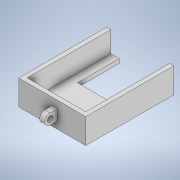
# Autodesk Inventor part: CAM04
Saved by Autodesk Inventor 2020.3 (Build 243373000, 373)
## iProperties
Created: 2021-05-24
Part Number: CAM04
Material: Generic
Document SubType Name: Modeling
Designer: patry
Density: 1 g/cm^3
Appearance: Default
Author: patry
Autodesk Inventor part; units mm, degrees
ref_plane "YZ Plane" through (0, 0, 0) normal (1, 0, 0) x (0, 1, 0)
ref_plane "XZ Plane" through (0, 0, 0) normal (0, 1, 0) x (-1, 0, 0)
ref_plane "XY Plane" through (0, 0, 0) normal (0, 0, 1) x (1, 0, 0)
sketch "Sketch1" plane through (0, 0, 0) normal (0, 1, 0) x (-1, 0, 0)
  line L0 (0, 0) -> (-32, 0)
  line L1 (-32, 0) -> (-32, 42)
  line L2 (-32, 42) -> (0, 42)
  line L3 (0, 42) -> (0, 0)
  dimension "d0" = 32
  dimension "d1" = 42
  constraints: 8 end point, 2 parallel, 1 horizontal, 1 perpendicular
  measures "d0" distance of L1.end L2.end
  measures "d1" distance of L0.end L1.end
extrude "Extrusion1" add sketch "Sketch1" along normal blind 2
sketch "Sketch2" plane through (0, 2, 0) normal (0, 1, 0) x (1, 0, 0)
  line L0 (0, -42) -> (32, -42) projected
  line L1 (0, 0) -> (32, 0)
  line L2 (32, 0) -> (32, -42)
  line L3 (32, -42) -> (0, -42)
  line L4 (0, -42) -> (0, 0)
  line L5 (0, 0) -> (0, -42) projected
  line L6 (0, 0) -> (2, 0)
  line L7 (2, 0) -> (2, -2)
  line L8 (2, -2) -> (0, -2)
  line L9 (0, -2) -> (0, 0)
  line L10 (32, -42) -> (30, -42)
  line L11 (30, -42) -> (30, -40)
  line L12 (30, -40) -> (32, -40)
  line L13 (32, -40) -> (32, -42)
  line L14 (30, -40) -> (2, -40)
  line L15 (2, -40) -> (2, -2)
  line L16 (2, -2) -> (30, -2)
  line L17 (30, -2) -> (30, -40)
  line L18 (32, -42) -> (32, 0) projected
  line L19 (30, -2) -> (32, -2)
  line L20 (32, -2) -> (32, 0)
  line L21 (32, 0) -> (30, 0)
  line L22 (30, 0) -> (30, -2)
  dimension "d4" = 2
  dimension "d5" = 2
  dimension "d6" = 2
  dimension "d7" = 2
  constraints: 40 end point, 10 parallel, 5 horizontal, 5 perpendicular
  measures "d4" distance of L7.end L8.end
  measures "d5" distance of L6.end L7.end
  measures "d6" distance of L11.end L12.end
  measures "d7" distance of L10.end L11.end
extrude "Extrusion2" add sketch "Sketch2" along normal blind 10 contours L4 L8 L15 L14 L11 L0 | L11 L12 L2 L0 | L4 L1 L7 L8 | L17 L19 L2 L12 | L22 L1 L2 L19
sketch "Sketch3" plane through (0, 2, 0) normal (0, 1, 0) x (1, 0, 0)
  line L0 (30, 0) -> (2, 0) projected
  line L1 (30, 0) -> (30, -40) projected
  line L2 (2, 0) -> (30, 0)
  line L3 (30, 0) -> (30, -40)
  line L4 (30, -40) -> (2, -40)
  line L5 (2, -40) -> (2, 0)
  line L6 (2, 0) -> (6, 0)
  line L7 (6, 0) -> (6, -4)
  line L8 (6, -4) -> (2, -4)
  line L9 (2, -4) -> (2, 0)
  line L10 (30, 0) -> (26, 0)
  line L11 (26, 0) -> (26, -4)
  line L12 (26, -4) -> (30, -4)
  line L13 (30, -4) -> (30, 0)
  line L14 (6, 0) -> (26, 0)
  line L15 (26, 0) -> (26, -20)
  line L16 (26, -20) -> (6, -20)
  line L17 (6, -20) -> (6, 0)
  point P0 (0, 0)
  dimension "d10" = 4
  dimension "d11" = 4
  dimension "d12" = 4
  dimension "d13" = 4
  dimension "d14" = 20
  dimension "d15" = 20
  constraints: 32 end point, 8 parallel, 4 horizontal, 4 perpendicular
  measures "d10" distance of L7.end L8.end
  measures "d11" distance of L6.end L7.end
  measures "d12" distance of L12.end L11.end
  measures "d13" distance of L11.end L10.end
  measures "d14" distance of L15.end L16.end
  measures "d15" distance of L14.end L15.end
extrude "Extrusion3" cut sketch "Sketch3" against normal through all contours L11 L15 L16 L17 L7 L0
sketch "Sketch4" plane through (0, 0, 42) normal (0, 0, 1) x (1, 0, 0)
  line L0 (2, 12) -> (0, 12) projected
  line L1 (32, 0) -> (26, 0) projected
  line L2 (0, 12) -> (32, 12)
  line L3 (32, 12) -> (32, 0)
  line L4 (32, 0) -> (0, 0)
  line L5 (0, 0) -> (0, 12)
  line L6 (0, 12) -> (13.5, 12)
  line L7 (13.5, 12) -> (13.5, 8.5)
  line L8 (13.5, 8.5) -> (0, 8.5)
  line L9 (0, 8.5) -> (0, 12)
  line L10 (13.5, 8.5) -> (18.5, 8.5)
  line L11 (18.5, 8.5) -> (18.5, 3.5)
  line L12 (18.5, 3.5) -> (13.5, 3.5)
  line L13 (13.5, 3.5) -> (13.5, 8.5)
  line L14 (18.5, 8.5) -> (16, 8.5)
  line L15 (16, 8.5) -> (16, 3.5)
  line L16 (16, 3.5) -> (18.5, 3.5)
  line L17 (18.5, 3.5) -> (18.5, 8.5)
  dimension "d18" = 13.5
  dimension "d19" = 3.5
  dimension "d20" = 5
  dimension "d21" = 5
  constraints: 32 end point, 8 parallel, 4 horizontal, 4 perpendicular, 1 midpoint
  measures "d18" distance of L7.end L8.end
  measures "d19" distance of L6.end L7.end
  measures "d20" distance of L11.end L12.end
  measures "d21" distance of L10.end L11.end
extrude "Extrusion4" add sketch "Sketch4" along normal blind 6 contours L10 L11 L12 L15
sketch "Sketch5" plane through (16, 3.5, 42) normal (-1, 0, 0) x (0, 0, 1)
  line L0 (6, 0) -> (6, 5) projected
  line L1 (6, 5) -> (3.5, 5)
  line L2 (3.5, 5) -> (3.5, 2.5)
  line L3 (3.5, 2.5) -> (6, 2.5)
  line L4 (6, 2.5) -> (6, 5)
  circle A0 centre (3.5, 2.5) radius 1.4
  point P0 (-42, -3.5)
  dimension "d24" = 2.5
  dimension "d25" = 2.5
  dimension "d26" = 2.8
  constraints: 8 end point, 2 parallel, 1 centre point, 1 coincident, 1 horizontal, 1 perpendicular
  measures "d24" distance of L3.end L2.end
  measures "d25" distance of L2.end L1.end
  measures "d26" diameter of A0
extrude "Extrusion5" cut sketch "Sketch5" against normal through all contours A0 L2 L3 | L3 L2 A0
fillet "Fillet1" radius 2.5 2 edges at (17.25, 8.5, 48) (17.25, 3.5, 48)
body "Solid1"
